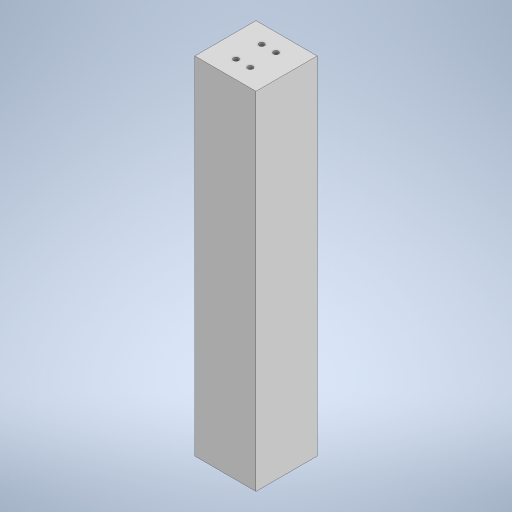
# Autodesk Inventor part: tower
Saved by Autodesk Inventor 2024 (Build 280153000, 153)
## iProperties
Created: 2023-11-02
Part Number: tower
Material: Generic
Document SubType Name: Modeling
Designer: dimademler
Density: 1 g/cm^3
Appearance: Default
Author: dimademler
Autodesk Inventor part; units mm, degrees
ref_plane "YZ Plane" through (0, 0, 0) normal (1, 0, 0) x (0, 1, 0)
ref_plane "XZ Plane" through (0, 0, 0) normal (0, 1, 0) x (-1, 0, 0)
ref_plane "XY Plane" through (0, 0, 0) normal (0, 0, 1) x (1, 0, 0)
sketch "Sketch1" plane through (0, 0, 0) normal (0, 1, 0) x (-1, 0, 0)
  line L0 (0, 0) -> (0, 76.2)
  line L1 (0, 76.2) -> (76.2, 76.2)
  line L2 (76.2, 76.2) -> (76.2, 0)
  line L3 (76.2, 0) -> (0, 0)
  dimension "d0" = 76.2
  dimension "d1" = 76.2
  constraints: 8 end point, 2 parallel, 1 perpendicular, 1 vertical
  measures "d0" distance of L0.start L0.end
  measures "d1" distance of L0.end L1.end
extrude "Extrusion1" add sketch "Sketch1" along normal blind 431.8
sketch "Sketch2" plane through (0, 431.8, 0) normal (0, 1, 0) x (1, 0, 0)
  line L0 (-76.2, -76.2) -> (0, -76.2) projected
  line L1 (-76.2, 0) -> (-76.2, -76.2) projected
  line L2 (0, 0) -> (-76.2, 0) projected
  line L3 (0, -76.2) -> (0, 0) projected
  line L4 (0, -38.1) -> (-76.2, -38.1) construction
  line L5 (-38.1, -38.1) -> (-38.1, -22.098) construction
  line L6 (-38.1, -22.098) -> (-46.99, -22.098) construction
  circle A0 centre (-46.99, -22.098) radius 2.032
  circle A1 centre (-29.21, -22.098) radius 2.032
  circle A2 centre (-46.99, -54.102) radius 2.032
  circle A3 centre (-29.21, -54.102) radius 2.032
  dimension "d4" = 16.002
  dimension "d5" = 8.89
  dimension "d6" = 4.064
  constraints: 6 end point, 4 centre point, 3 midpoint, 3 symmetric about line, 1 coincident, 1 perpendicular, 1 vertical, 3 other
  measures "d4" distance of L5.start L5.end
  measures "d5" distance of L5.end L6.end
  measures "d6" diameter of A0
hole "Hole1" at (-46.99, 431.8, 54.102) at (-29.21, 431.8, 54.102) at (-29.21, 431.8, 22.098) at (-46.99, 431.8, 22.098) direction (0, -1, 0) diameter 6.35 depth 25.4 tip angle 118
body "Solid1"
